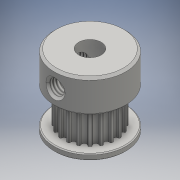
# Autodesk Inventor part: GT2_Pulley
Saved by Autodesk Inventor 2016 (Build 200138000, 138)
## iProperties
Created: 2021-12-07
Part Number: GT2_Pulley
Material: Generic
Document SubType Name: Modeling
Designer: Muntean Ioan
Density: 1 g/cm^3
Appearance: Default
Author: Muntean Ioan
Autodesk Inventor part; units mm, degrees
ref_plane "YZ Plane" through (0, 0, 0) normal (1, 0, 0) x (0, 1, 0)
ref_plane "XZ Plane" through (0, 0, 0) normal (0, 1, 0) x (-1, 0, 0)
ref_plane "XY Plane" through (0, 0, 0) normal (0, 0, 1) x (1, 0, 0)
sketch "Sketch1" plane through (0, 0, 0) normal (0, 1, 0) x (-1, 0, 0)
  line L0 (0, 0) -> (0, 15)
  line L1 (0, 0) -> (15, 0) construction
  line L2 (2.5, 0) -> (8, 0)
  line L3 (8, 0) -> (8, 1.3)
  line L4 (8, 1.3) -> (6, 1.3)
  line L5 (6, 1.3) -> (6, 8.6)
  line L6 (6, 8.6) -> (7.975, 8.6)
  line L7 (7.975, 8.6) -> (7.975, 16)
  line L8 (7.975, 16) -> (2.5, 16)
  line L9 (2.5, 16) -> (2.5, 0)
  dimension "d0" = 15
  dimension "d1" = 90
  dimension "d2" = 8
  dimension "d3" = 1.3
  dimension "d4" = 7.3
  dimension "d5" = 16
  dimension "d6" = 7.4
  dimension "d7" = 7.975
  dimension "d8" = 6
  dimension "d9" = 2.5
  constraints: 20 end point, 6 perpendicular, 3 vertical, 2 point on line, 1 horizontal
  measures "d0" distance of L0.start L0.end
  measures "d1" angle of L1 L0
  measures "d2" distance between parallel lines of L0 L3
  measures "d3" distance of L2.end L3.end
  measures "d4" distance of L4.end L5.end
  measures "d5" distance of L8.end L2.start
  measures "d6" distance of L6.end L7.end
  measures "d7" distance between parallel lines of L7 L0
  measures "d8" distance between parallel lines of L0 L5
  measures "d9" distance between parallel lines of L0 L9
revolve "Revolution1" add sketch "Sketch1" angle 360 about axis through (0, 0, 0) along (0, 0, 1)
sketch "Sketch3" plane through (0, 0, 1.3) normal (0, 0, 1) x (1, 0, 0)
  line L0 (-1.0664, 6.5842) -> (7.3715, 6.5842) construction
  line L1 (-3.036, 5.9542) -> (7.6612, 5.9542) construction
  line L2 (0, 8) -> (0, 2.4044) construction
  line L3 (-3.1549, 5.2042) -> (7.6437, 5.2042) construction
  line L4 (0.4, 6.6743) -> (0.4, 2.3928) construction
  arc A0 (-0.5915, 5.8237) -> (-0.7402, 5.9542) centre (-0.7402, 5.8042) ccw
  arc A1 (-0.4989, 5.516) -> (0, 5.2042) centre (0, 5.7592) ccw
  line L5 (-1, 6.8691) -> (-1, 2.1684) construction
  arc A2 (-0.5915, 5.8237) -> (-0.4989, 5.516) centre (0.4, 5.9542) ccw
  line L6 (-0.7402, 5.9542) -> (-1, 5.9542)
  arc A3 (0.7402, 5.9542) -> (0.5915, 5.8237) centre (0.7402, 5.8042) ccw
  arc A4 (0, 5.2042) -> (0.4989, 5.516) centre (0, 5.7592) ccw
  arc A5 (0.4989, 5.516) -> (0.5915, 5.8237) centre (-0.4, 5.9542) ccw
  line L7 (0.7402, 5.9542) -> (1, 5.9542)
  line L8 (1, 2.0244) -> (1, 7.1901) construction
  arc A6 (0.7927, 5.1587) -> (0.7266, 5.4347) centre (0.7124, 5.2854) ccw construction
  line L9 (0.7266, 5.4347) -> (0.5155, 5.4415) construction
  circle A7 centre (0, 0) radius 2.5 construction
  circle A8 centre (0, 0) radius 6 construction
  circle A9 centre (0, 0) radius 8 construction
  line L10 (1, 5.9542) -> (1, 6.4854) construction
  line L11 (1, 5.9542) -> (1, 6.2198)
  line L12 (1, 6.2198) -> (-1, 6.2198)
  line L13 (-1, 5.9542) -> (-1, 6.2198)
  dimension "d27" = 1.38
  dimension "d28" = 0.75
  dimension "d31" = 0.4
  dimension "d33" = 0.555
  dimension "d34" = 1
  dimension "d36" = 1
  dimension "d38" = 0.15
  dimension "d39" = 0.63
  dimension "d40" = 2
  dimension "d43" = 0.15
  dimension "d45" = 0.5196
  constraints: 28 end point, 16 point on circle, 10 point on line, 7 centre point, 6 symmetric about line, 4 vertical, 3 horizontal, 3 tangent, 1 collinear, 1 midpoint, 1 perpendicular, 1 vertical alignment, 4 other
  measures "d27" distance between parallel lines of L3 L0
  measures "d28" distance between parallel lines of L1 L3
  measures "d31" distance between parallel lines of L4 L2
  measures "d33" radius of A1
  measures "d34" distance between parallel lines of L2 L5
  measures "d36" radius of A2
  measures "d38" radius of A0
  measures "d39" distance between parallel lines of L0 L1
  measures "d40" distance between parallel lines of L8 L5
  measures "d43" radius of A6
  measures "d45" distance of L9.start L7.start
extrude "Extrusion1" cut sketch "Sketch3" along normal up to surface (7.3 mm away)
pattern_circular "Circular Pattern1" count 20 over 360 about axis through (0, 0, 0.65) along (0, 0, -1) of "Extrusion1"
chamfer "Chamfer1" distance 0.5 angle 45 2 edges at (7.975, 0, 8.6) (7.975, 0, 16)
sketch "Sketch4" plane through (0, 0, 0) normal (0, 1, 0) x (-1, 0, 0)
  line L0 (-7.475, 16) -> (7.475, 16) construction
  line L1 (7.475, 8.6) -> (-7.475, 8.6) construction
  circle A0 centre (0, 12.3) radius 1.65
  point P0 (0, 0)
  dimension "d54" = 3.3
  dimension "d55" = 7.4
  dimension "d56" = 3.7
  constraints: 1 centre point
  measures "d54" diameter of A0
  measures "d55" distance between parallel lines of L1 L0
  measures "d56" distance from line of A0.centre L1
extrude "Extrusion2" cut sketch "Sketch4" against normal blind 10
chamfer "Chamfer2" distance 0.5 angle 45 1 edges at (1.65, -7.8024, 12.3011)
thread "Thread1" size "M4x0.7" class "6H" standard "ISO Metric profile" full length
pattern_circular "Circular Pattern2" count 2 over 90 about axis through (0, 0, 12.3) along (0, 0, -1) of "Extrusion2", "Chamfer2"
chamfer "Chamfer3" distance 0.2 angle 45 2 edges at (8, 0, 1.3) (8, 0, 0)
body "Solid1"
